Autodesk Fusion 360 part; units mm, degrees
(part 10 of 13)
  line L8044 (144.1, -138.589) -> (144.278, -138.571)
  line L8045 (144.602, -140.099) -> (144.433, -140.154)
  line L8046 (143.779, -138.74) -> (143.931, -138.647)
  line L8047 (118.974, -133.265) -> (118.977, -133.268)
  line L8048 (121.742, -140.099) -> (121.573, -140.154)
  line L8049 (119.499, -138.874) -> (119.593, -139.025)
  line L8050 (118.238, -139.859) -> (118.146, -139.706)
  line L8051 (118.252, -138.865) -> (118.379, -138.74)
  line L8052 (118.747, -133.387) -> (117.468, -132.108)
  line L8053 (117.291, -132.155) -> (117.168, -132.135)
  line L8054 (121.573, -140.154) -> (121.395, -140.17)
  line L8055 (122.212, -139.371) -> (122.212, -139.393)
  line L8056 (118.747, -138.584) -> (118.747, -133.387)
  line L8057 (119.356, -140.008) -> (119.202, -140.099)
  line L8058 (116.891, -131.755) -> (116.911, -131.631)
  line L8059 (119.223, -138.652) -> (119.373, -138.747)
  line L8060 (117.056, -131.431) -> (117.168, -131.374)
  line L8061 (117.415, -132.135) -> (117.291, -132.155)
  line L8062 (118.7, -138.589) -> (118.747, -138.584)
  line L8063 (119.485, -139.885) -> (119.356, -140.008)
  line L8064 (119.672, -139.371) -> (119.672, -139.393)
  line L8065 (118.072, -139.359) -> (118.094, -139.182)
  line L8066 (119.652, -139.193) -> (119.672, -139.371)
  line L8067 (119.033, -140.154) -> (118.855, -140.17)
  line L8068 (116.968, -131.52) -> (117.056, -131.431)
  line L8069 (121.595, -138.592) -> (121.763, -138.652)
  line L8070 (119.373, -138.747) -> (119.499, -138.874)
  line L8071 (119.202, -140.099) -> (119.033, -140.154)
  line L8072 (121.218, -140.147) -> (121.051, -140.085)
  line L8073 (122.124, -139.736) -> (122.025, -139.885)
  line L8074 (116.911, -131.878) -> (116.891, -131.755)
  line L8075 (118.379, -138.74) -> (118.531, -138.647)
  line L8076 (120.902, -139.987) -> (120.778, -139.859)
  line L8077 (117.168, -132.135) -> (117.056, -132.078)
  line L8078 (118.997, -133.336) -> (118.997, -138.585)
  line L8079 (118.997, -138.585) -> (119.055, -138.592)
  line L8080 (121.763, -138.652) -> (121.913, -138.747)
  line L8081 (119.055, -138.592) -> (119.223, -138.652)
  line L8082 (119.647, -139.57) -> (119.584, -139.736)
  line L8083 (121.913, -138.747) -> (122.039, -138.874)
  line L8084 (121.896, -140.008) -> (121.742, -140.099)
  line L8085 (117.291, -131.355) -> (117.415, -131.374)
  line L8086 (117.468, -132.108) -> (117.415, -132.135)
  line L8087 (118.362, -139.987) -> (118.238, -139.859)
  line L8088 (121.051, -140.085) -> (120.902, -139.987)
  line L8089 (117.168, -131.374) -> (117.291, -131.355)
  line L8090 (122.039, -138.874) -> (122.133, -139.025)
  line L8091 (121.395, -140.17) -> (121.218, -140.147)
  line L8092 (116.911, -131.631) -> (116.968, -131.52)
  line L8093 (122.187, -139.57) -> (122.124, -139.736)
  line L8094 (122.212, -139.393) -> (122.187, -139.57)
  line L8095 (119.584, -139.736) -> (119.485, -139.885)
  line L8096 (136.835, -138.592) -> (137.003, -138.652)
  line L8097 (120.629, -139.537) -> (120.612, -139.359)
  line L8098 (121.24, -138.589) -> (121.418, -138.571)
  line L8099 (136.813, -140.154) -> (136.635, -140.17)
  line L8100 (123.152, -139.359) -> (123.174, -139.182)
  line L8101 (123.318, -139.859) -> (123.226, -139.706)
  line L8102 (136.458, -140.147) -> (136.291, -140.085)
  line L8103 (123.174, -139.182) -> (123.235, -139.015)
  line L8104 (124.135, -138.592) -> (124.303, -138.652)
  line L8105 (135.926, -139.706) -> (135.869, -139.537)
  line L8106 (124.664, -139.736) -> (124.565, -139.885)
  line L8107 (137.364, -139.736) -> (137.265, -139.885)
  line L8108 (136.018, -139.859) -> (135.926, -139.706)
  line L8109 (122.192, -139.193) -> (122.212, -139.371)
  line L8110 (137.279, -138.874) -> (137.373, -139.025)
  line L8111 (123.169, -139.537) -> (123.152, -139.359)
  line L8112 (135.935, -139.015) -> (136.032, -138.865)
  line L8113 (124.113, -140.154) -> (123.935, -140.17)
  line L8114 (124.752, -139.393) -> (124.727, -139.57)
  line L8115 (120.612, -139.359) -> (120.634, -139.182)
  line L8116 (137.432, -139.193) -> (137.452, -139.371)
  line L8117 (120.634, -139.182) -> (120.695, -139.015)
  line L8118 (137.265, -139.885) -> (137.136, -140.008)
  line L8119 (123.235, -139.015) -> (123.332, -138.865)
  line L8120 (124.673, -139.025) -> (124.732, -139.193)
  line L8121 (120.792, -138.865) -> (120.919, -138.74)
  line L8122 (137.373, -139.025) -> (137.432, -139.193)
  line L8123 (137.136, -140.008) -> (136.982, -140.099)
  line L8124 (137.452, -139.393) -> (137.427, -139.57)
  line L8125 (137.003, -138.652) -> (137.153, -138.747)
  line L8126 (120.686, -139.706) -> (120.629, -139.537)
  line L8127 (136.982, -140.099) -> (136.813, -140.154)
  line L8128 (136.142, -139.987) -> (136.018, -139.859)
  line L8129 (137.153, -138.747) -> (137.279, -138.874)
  line L8130 (117.056, -132.078) -> (116.968, -131.99)
  line L8131 (137.427, -139.57) -> (137.364, -139.736)
  line L8132 (120.778, -139.859) -> (120.686, -139.706)
  line L8133 (137.452, -139.371) -> (137.452, -139.393)
  line L8134 (116.968, -131.99) -> (116.911, -131.878)
  line L8135 (120.919, -138.74) -> (121.071, -138.647)
  line L8136 (122.025, -139.885) -> (121.896, -140.008)
  line L8137 (121.418, -138.571) -> (121.595, -138.592)
  line L8138 (122.133, -139.025) -> (122.192, -139.193)
  line L8139 (135.869, -139.537) -> (135.852, -139.359)
  line L8140 (136.291, -140.085) -> (136.142, -139.987)
  line L8141 (121.071, -138.647) -> (121.24, -138.589)
  line L8142 (136.635, -140.17) -> (136.458, -140.147)
  line L8143 (120.695, -139.015) -> (120.792, -138.865)
  line L8144 (124.303, -138.652) -> (124.453, -138.747)
  line L8145 (127.119, -138.874) -> (127.213, -139.025)
  line L8146 (125.766, -139.706) -> (125.709, -139.537)
  line L8147 (124.453, -138.747) -> (124.579, -138.874)
  line L8148 (124.579, -138.874) -> (124.673, -139.025)
  line L8149 (136.658, -138.571) -> (136.835, -138.592)
  line L8150 (123.442, -139.987) -> (123.318, -139.859)
  line L8151 (124.752, -139.371) -> (124.752, -139.393)
  line L8152 (127.204, -139.736) -> (127.105, -139.885)
  line L8153 (127.292, -139.393) -> (127.267, -139.57)
  line L8154 (126.843, -138.652) -> (126.993, -138.747)
  line L8155 (136.159, -138.74) -> (136.311, -138.647)
  line L8156 (135.852, -139.359) -> (135.874, -139.182)
  line L8157 (125.999, -138.74) -> (126.151, -138.647)
  line L8158 (123.459, -138.74) -> (123.611, -138.647)
  line L8159 (126.822, -140.099) -> (126.653, -140.154)
  line L8160 (126.653, -140.154) -> (126.475, -140.17)
  line L8161 (126.151, -138.647) -> (126.32, -138.589)
  line L8162 (126.475, -140.17) -> (126.298, -140.147)
  line L8163 (136.48, -138.589) -> (136.658, -138.571)
  line L8164 (136.311, -138.647) -> (136.48, -138.589)
  line L8165 (123.935, -140.17) -> (123.758, -140.147)
  line L8166 (124.282, -140.099) -> (124.113, -140.154)
  line L8167 (136.032, -138.865) -> (136.159, -138.74)
  line L8168 (123.758, -140.147) -> (123.591, -140.085)
  line L8169 (125.692, -139.359) -> (125.714, -139.182)
  line L8170 (125.872, -138.865) -> (125.999, -138.74)
  line L8171 (127.272, -139.193) -> (127.292, -139.371)
  line L8172 (126.131, -140.085) -> (125.982, -139.987)
  line L8173 (123.226, -139.706) -> (123.169, -139.537)
  line L8174 (124.727, -139.57) -> (124.664, -139.736)
  line L8175 (123.332, -138.865) -> (123.459, -138.74)
  line L8176 (126.976, -140.008) -> (126.822, -140.099)
  line L8177 (125.714, -139.182) -> (125.775, -139.015)
  line L8178 (124.436, -140.008) -> (124.282, -140.099)
  line L8179 (123.611, -138.647) -> (123.78, -138.589)
  line L8180 (126.298, -140.147) -> (126.131, -140.085)
  line L8181 (125.982, -139.987) -> (125.858, -139.859)
  line L8182 (125.858, -139.859) -> (125.766, -139.706)
  line L8183 (125.775, -139.015) -> (125.872, -138.865)
  line L8184 (124.732, -139.193) -> (124.752, -139.371)
  line L8185 (127.292, -139.371) -> (127.292, -139.393)
  line L8186 (126.675, -138.592) -> (126.843, -138.652)
  line L8187 (123.958, -138.571) -> (124.135, -138.592)
  line L8188 (135.874, -139.182) -> (135.935, -139.015)
  line L8189 (124.565, -139.885) -> (124.436, -140.008)
  line L8190 (123.78, -138.589) -> (123.958, -138.571)
  line L8191 (123.591, -140.085) -> (123.442, -139.987)
  line L8192 (115.822, -139.987) -> (115.698, -139.859)
  line L8193 (131.755, -138.592) -> (131.923, -138.652)
  line L8194 (115.698, -139.859) -> (115.606, -139.706)
  line L8195 (116.493, -140.154) -> (116.315, -140.17)
  line L8196 (126.993, -138.747) -> (127.119, -138.874)
  line L8197 (115.839, -138.74) -> (115.991, -138.647)
  line L8198 (116.338, -138.571) -> (116.515, -138.592)
  line L8199 (116.662, -140.099) -> (116.493, -140.154)
  line L8200 (125.709, -139.537) -> (125.692, -139.359)
  line L8201 (129.215, -138.592) -> (129.383, -138.652)
  line L8202 (116.515, -138.592) -> (116.683, -138.652)
  line L8203 (116.683, -138.652) -> (116.833, -138.747)
  line L8204 (116.315, -140.17) -> (116.138, -140.147)
  line L8205 (115.712, -138.865) -> (115.839, -138.74)
  line L8206 (127.267, -139.57) -> (127.204, -139.736)
  line L8207 (127.105, -139.885) -> (126.976, -140.008)
  line L8208 (126.498, -138.571) -> (126.675, -138.592)
  line L8209 (115.532, -139.359) -> (115.554, -139.182)
  line L8210 (117.112, -139.193) -> (117.132, -139.371)
  line L8211 (115.971, -140.085) -> (115.822, -139.987)
  line L8212 (116.833, -138.747) -> (116.959, -138.874)
  line L8213 (115.615, -139.015) -> (115.712, -138.865)
  line L8214 (115.549, -139.537) -> (115.532, -139.359)
  line L8215 (126.32, -138.589) -> (126.498, -138.571)
  line L8216 (115.991, -138.647) -> (116.16, -138.589)
  line L8217 (116.16, -138.589) -> (116.338, -138.571)
  line L8218 (129.753, -139.025) -> (129.812, -139.193)
  line L8219 (115.554, -139.182) -> (115.615, -139.015)
  line L8220 (117.132, -139.371) -> (117.132, -139.393)
  line L8221 (128.398, -139.859) -> (128.306, -139.706)
  line L8222 (128.315, -139.015) -> (128.412, -138.865)
  line L8223 (115.606, -139.706) -> (115.549, -139.537)
  line L8224 (117.044, -139.736) -> (116.945, -139.885)
  line L8225 (116.945, -139.885) -> (116.816, -140.008)
  line L8226 (116.816, -140.008) -> (116.662, -140.099)
  line L8227 (117.132, -139.393) -> (117.107, -139.57)
  line L8228 (129.193, -140.154) -> (129.015, -140.17)
  line L8229 (129.659, -138.874) -> (129.753, -139.025)
  line L8230 (117.107, -139.57) -> (117.044, -139.736)
  line L8231 (127.213, -139.025) -> (127.272, -139.193)
  line L8232 (129.744, -139.736) -> (129.645, -139.885)
  line L8233 (116.959, -138.874) -> (117.053, -139.025)
  line L8234 (128.691, -138.647) -> (128.86, -138.589)
  line L8235 (117.053, -139.025) -> (117.112, -139.193)
  line L8236 (128.86, -138.589) -> (129.038, -138.571)
  line L8237 (129.832, -139.393) -> (129.807, -139.57)
  line L8238 (116.138, -140.147) -> (115.971, -140.085)
  line L8239 (129.038, -138.571) -> (129.215, -138.592)
  line L8240 (131.555, -140.17) -> (131.378, -140.147)
  line L8241 (130.855, -139.015) -> (130.952, -138.865)
  line L8242 (132.199, -138.874) -> (132.293, -139.025)
  line L8243 (139.693, -138.747) -> (139.819, -138.874)
  line L8244 (132.284, -139.736) -> (132.185, -139.885)
  line L8245 (139.913, -139.025) -> (139.972, -139.193)
  line L8246 (129.015, -140.17) -> (128.838, -140.147)
  line L8247 (132.293, -139.025) -> (132.352, -139.193)
  line L8248 (129.812, -139.193) -> (129.832, -139.371)
  line L8249 (128.412, -138.865) -> (128.539, -138.74)
  line L8250 (128.232, -139.359) -> (128.254, -139.182)
  line L8251 (130.789, -139.537) -> (130.772, -139.359)
  line L8252 (128.249, -139.537) -> (128.232, -139.359)
  line L8253 (130.772, -139.359) -> (130.794, -139.182)
  line L8254 (131.902, -140.099) -> (131.733, -140.154)
  line L8255 (131.378, -140.147) -> (131.211, -140.085)
  line L8256 (129.645, -139.885) -> (129.516, -140.008)
  line L8257 (129.362, -140.099) -> (129.193, -140.154)
  line L8258 (139.992, -139.371) -> (139.992, -139.393)
  line L8259 (129.516, -140.008) -> (129.362, -140.099)
  line L8260 (132.372, -139.371) -> (132.372, -139.393)
  line L8261 (131.733, -140.154) -> (131.555, -140.17)
  line L8262 (128.671, -140.085) -> (128.522, -139.987)
  line L8263 (129.807, -139.57) -> (129.744, -139.736)
  line L8264 (128.306, -139.706) -> (128.249, -139.537)
  line L8265 (128.254, -139.182) -> (128.315, -139.015)
  line L8266 (139.543, -138.652) -> (139.693, -138.747)
  line L8267 (129.383, -138.652) -> (129.533, -138.747)
  line L8268 (131.923, -138.652) -> (132.073, -138.747)
  line L8269 (131.062, -139.987) -> (130.938, -139.859)
  line L8270 (131.231, -138.647) -> (131.4, -138.589)
  line L8271 (132.185, -139.885) -> (132.056, -140.008)
  line L8272 (132.352, -139.193) -> (132.372, -139.371)
  line L8273 (139.819, -138.874) -> (139.913, -139.025)
  line L8274 (130.846, -139.706) -> (130.789, -139.537)
  line L8275 (139.375, -138.592) -> (139.543, -138.652)
  line L8276 (132.347, -139.57) -> (132.284, -139.736)
  line L8277 (129.832, -139.371) -> (129.832, -139.393)
  line L8278 (128.522, -139.987) -> (128.398, -139.859)
  line L8279 (131.578, -138.571) -> (131.755, -138.592)
  line L8280 (128.838, -140.147) -> (128.671, -140.085)
  line L8281 (128.539, -138.74) -> (128.691, -138.647)
  line L8282 (132.073, -138.747) -> (132.199, -138.874)
  line L8283 (131.4, -138.589) -> (131.578, -138.571)
  line L8284 (129.533, -138.747) -> (129.659, -138.874)
  line L8285 (131.079, -138.74) -> (131.231, -138.647)
  line L8286 (132.056, -140.008) -> (131.902, -140.099)
  line L8287 (132.372, -139.393) -> (132.347, -139.57)
  line L8288 (139.522, -140.099) -> (139.353, -140.154)
  line L8289 (142.359, -138.874) -> (142.453, -139.025)
  line L8290 (139.198, -138.571) -> (139.375, -138.592)
  line L8291 (142.512, -139.193) -> (142.532, -139.371)
  line L8292 (134.887, -139.57) -> (134.824, -139.736)
  line L8293 (142.062, -140.099) -> (141.893, -140.154)
  line L8294 (141.239, -138.74) -> (141.391, -138.647)
  line L8295 (140.949, -139.537) -> (140.932, -139.359)
  line L8296 (142.216, -140.008) -> (142.062, -140.099)
  line L8297 (138.414, -139.182) -> (138.475, -139.015)
  line L8298 (142.507, -139.57) -> (142.444, -139.736)
  line L8299 (138.558, -139.859) -> (138.466, -139.706)
  line L8300 (141.006, -139.706) -> (140.949, -139.537)
  line L8301 (141.915, -138.592) -> (142.083, -138.652)
  line L8302 (130.952, -138.865) -> (131.079, -138.74)
  line L8303 (142.532, -139.371) -> (142.532, -139.393)
  line L8304 (139.992, -139.393) -> (139.967, -139.57)
  line L8305 (138.851, -138.647) -> (139.02, -138.589)
  line L8306 (138.466, -139.706) -> (138.409, -139.537)
  line L8307 (142.444, -139.736) -> (142.345, -139.885)
  line L8308 (138.475, -139.015) -> (138.572, -138.865)
  line L8309 (138.831, -140.085) -> (138.682, -139.987)
  line L8310 (130.938, -139.859) -> (130.846, -139.706)
  line L8311 (139.175, -140.17) -> (138.998, -140.147)
  line L8312 (140.932, -139.359) -> (140.954, -139.182)
  line L8313 (142.083, -138.652) -> (142.233, -138.747)
  line L8314 (139.967, -139.57) -> (139.904, -139.736)
  line L8315 (142.345, -139.885) -> (142.216, -140.008)
  line L8316 (134.596, -140.008) -> (134.442, -140.099)
  line L8317 (131.211, -140.085) -> (131.062, -139.987)
  line L8318 (138.699, -138.74) -> (138.851, -138.647)
  line L8319 (142.532, -139.393) -> (142.507, -139.57)
  line L8320 (134.442, -140.099) -> (134.273, -140.154)
  line L8321 (139.02, -138.589) -> (139.198, -138.571)
  line L8322 (141.538, -140.147) -> (141.371, -140.085)
  line L8323 (139.972, -139.193) -> (139.992, -139.371)
  line L8324 (142.453, -139.025) -> (142.512, -139.193)
  line L8325 (138.682, -139.987) -> (138.558, -139.859)
  line L8326 (139.805, -139.885) -> (139.676, -140.008)
  line L8327 (130.794, -139.182) -> (130.855, -139.015)
  line L8328 (139.353, -140.154) -> (139.175, -140.17)
  line L8329 (142.233, -138.747) -> (142.359, -138.874)
  line L8330 (139.676, -140.008) -> (139.522, -140.099)
  line L8331 (138.998, -140.147) -> (138.831, -140.085)
  line L8332 (139.904, -139.736) -> (139.805, -139.885)
  line L8333 (138.392, -139.359) -> (138.414, -139.182)
  line L8334 (138.572, -138.865) -> (138.699, -138.74)
  line L8335 (138.409, -139.537) -> (138.392, -139.359)
  line L8336 (141.715, -140.17) -> (141.538, -140.147)
  line L8337 (134.273, -140.154) -> (134.095, -140.17)
  line L8338 (133.751, -140.085) -> (133.602, -139.987)
  line L8339 (134.095, -140.17) -> (133.918, -140.147)
  line L8340 (147.533, -139.025) -> (147.592, -139.193)
  line L8341 (141.391, -138.647) -> (141.56, -138.589)
  line L8342 (141.56, -138.589) -> (141.738, -138.571)
  line L8343 (134.295, -138.592) -> (134.463, -138.652)
  line L8344 (147.142, -140.099) -> (146.973, -140.154)
  line L8345 (147.425, -139.885) -> (147.296, -140.008)
  line L8346 (146.995, -138.592) -> (147.163, -138.652)
  line L8347 (134.725, -139.885) -> (134.596, -140.008)
  line L8348 (134.912, -139.393) -> (134.887, -139.57)
  line L8349 (141.098, -139.859) -> (141.006, -139.706)
  line L8350 (146.973, -140.154) -> (146.795, -140.17)
  line L8351 (146.795, -140.17) -> (146.618, -140.147)
  line L8352 (133.312, -139.359) -> (133.334, -139.182)
  line L8353 (141.222, -139.987) -> (141.098, -139.859)
  line L8354 (147.587, -139.57) -> (147.524, -139.736)
  line L8355 (141.738, -138.571) -> (141.915, -138.592)
  line L8356 (134.833, -139.025) -> (134.892, -139.193)
  line L8357 (133.334, -139.182) -> (133.395, -139.015)
  line L8358 (134.613, -138.747) -> (134.739, -138.874)
  line L8359 (141.015, -139.015) -> (141.112, -138.865)
  line L8360 (147.296, -140.008) -> (147.142, -140.099)
  line L8361 (146.618, -140.147) -> (146.451, -140.085)
  line L8362 (147.524, -139.736) -> (147.425, -139.885)
  line L8363 (133.94, -138.589) -> (134.118, -138.571)
  line L8364 (133.395, -139.015) -> (133.492, -138.865)
  line L8365 (141.112, -138.865) -> (141.239, -138.74)
  line L8366 (147.439, -138.874) -> (147.533, -139.025)
  line L8367 (147.313, -138.747) -> (147.439, -138.874)
  line L8368 (133.478, -139.859) -> (133.386, -139.706)
  line L8369 (141.893, -140.154) -> (141.715, -140.17)
  line L8370 (134.463, -138.652) -> (134.613, -138.747)
  line L8371 (147.612, -139.371) -> (147.612, -139.393)
  line L8372 (134.118, -138.571) -> (134.295, -138.592)
  line L8373 (140.954, -139.182) -> (141.015, -139.015)
  line L8374 (134.892, -139.193) -> (134.912, -139.371)
  line L8375 (141.371, -140.085) -> (141.222, -139.987)
  line L8376 (134.739, -138.874) -> (134.833, -139.025)
  line L8377 (133.771, -138.647) -> (133.94, -138.589)
  line L8378 (134.824, -139.736) -> (134.725, -139.885)
  line L8379 (133.386, -139.706) -> (133.329, -139.537)
  line L8380 (133.619, -138.74) -> (133.771, -138.647)
  line L8381 (133.492, -138.865) -> (133.619, -138.74)
  line L8382 (147.163, -138.652) -> (147.313, -138.747)
  line L8383 (134.912, -139.371) -> (134.912, -139.393)
  line L8384 (143.75, -124.929) -> (143.732, -124.943)
  line L8385 (146.086, -122.026) -> (146.029, -121.857)
  line L8386 (143.726, -124.947) -> (143.721, -124.951)
  line L8387 (146.319, -138.74) -> (146.471, -138.647)
  line L8388 (147.612, -139.393) -> (147.587, -139.57)
  line L8389 (105.027, -122.529) -> (107.214, -124.716)
  line L8390 (146.818, -138.571) -> (146.995, -138.592)
  line L8391 (105.744, -119.532) -> (105.691, -119.505)
  line L8392 (146.64, -138.589) -> (146.818, -138.571)
  line L8393 (146.471, -138.647) -> (146.64, -138.589)
  line L8394 (107.214, -124.716) -> (143.61, -124.716)
  line L8395 (105.867, -119.551) -> (105.744, -119.532)
  line L8396 (106.191, -119.387) -> (106.102, -119.475)
  line L8397 (147.592, -139.193) -> (147.612, -139.371)
  line L8398 (106.248, -119.275) -> (106.191, -119.387)
  line L8399 (105.991, -118.771) -> (106.102, -118.828)
  line L8400 (146.012, -139.359) -> (146.034, -139.182)
  line L8401 (106.267, -119.151) -> (106.248, -119.275)
  line L8402 (106.248, -119.028) -> (106.267, -119.151)
  line L8403 (133.918, -140.147) -> (133.751, -140.085)
  line L8404 (146.086, -139.706) -> (146.029, -139.537)
  line L8405 (146.166, -122.159) -> (146.086, -122.026)
  line L8406 (146.034, -139.182) -> (146.095, -139.015)
  line L8407 (146.178, -139.859) -> (146.086, -139.706)
  line L8408 (146.029, -121.857) -> (146.012, -121.679)
  line L8409 (106.102, -119.475) -> (105.991, -119.532)
  line L8410 (105.027, -120.168) -> (105.027, -122.529)
  line L8411 (146.451, -122.405) -> (146.345, -122.335)
  line L8412 (146.64, -120.909) -> (146.818, -120.891)
  line L8413 (106.102, -118.828) -> (106.191, -118.916)
  line L8414 (105.991, -119.532) -> (105.867, -119.551)
  line L8415 (146.192, -121.185) -> (146.319, -121.06)
  line L8416 (146.029, -139.537) -> (146.012, -139.359)
  line L8417 (146.095, -139.015) -> (146.192, -138.865)
  line L8418 (146.451, -140.085) -> (146.302, -139.987)
  line L8419 (143.61, -124.716) -> (146.166, -122.159)
  line L8420 (147.612, -121.713) -> (147.587, -121.89)
  line L8421 (146.618, -122.467) -> (146.451, -122.405)
  line L8422 (133.602, -139.987) -> (133.478, -139.859)
  line L8423 (146.302, -139.987) -> (146.178, -139.859)
  line L8424 (147.612, -121.691) -> (147.612, -121.713)
  line L8425 (105.691, -119.505) -> (105.027, -120.168)
  line L8426 (133.329, -139.537) -> (133.312, -139.359)
  line L8427 (146.192, -138.865) -> (146.319, -138.74)
  line L8428 (106.191, -118.916) -> (106.248, -119.028)
  line L8429 (146.795, -122.49) -> (146.618, -122.467)
  line L8430 (146.319, -121.06) -> (146.471, -120.967)
  line L8431 (147.587, -121.89) -> (147.524, -122.056)
  line L8432 (104.78, -120.09) -> (104.781, -120.087)
  line L8433 (143.729, -124.946) -> (143.726, -124.947)
  line L8434 (107.127, -124.961) -> (107.101, -124.944)
  line L8435 (143.626, -122.159) -> (143.546, -122.026)
  line L8436 (107.074, -124.929) -> (104.814, -122.669)
  line L8437 (104.777, -122.58) -> (104.777, -120.117)
  line L8438 (146.034, -121.502) -> (146.095, -121.335)
  line L8439 (146.012, -121.679) -> (146.034, -121.502)
  line L8440 (104.814, -120.028) -> (105.514, -119.328)
  line L8441 (143.721, -124.951) -> (143.691, -124.957)
  line L8442 (147.592, -121.513) -> (147.612, -121.691)
  line L8443 (147.142, -122.419) -> (146.973, -122.474)
  line L8444 (147.163, -120.972) -> (147.313, -121.067)
  line L8445 (143.546, -122.026) -> (143.489, -121.857)
  line L8446 (105.544, -118.916) -> (105.632, -118.828)
  line L8447 (104.814, -122.669) -> (104.8, -122.651)
  line L8448 (104.796, -122.645) -> (104.792, -122.64)
  line L8449 (107.136, -124.963) -> (107.133, -124.962)
  line L8450 (146.345, -122.335) -> (143.75, -124.929)
  line L8451 (146.818, -120.891) -> (146.995, -120.912)
  line L8452 (147.439, -121.194) -> (147.533, -121.345)
  line L8453 (146.471, -120.967) -> (146.64, -120.909)
  line L8454 (104.792, -122.64) -> (104.786, -122.61)
  line L8455 (104.799, -120.055) -> (104.814, -120.028)
  line L8456 (146.995, -120.912) -> (147.163, -120.972)
  line L8457 (147.533, -121.345) -> (147.592, -121.513)
  line L8458 (143.732, -124.943) -> (143.729, -124.946)
  line L8459 (105.744, -118.771) -> (105.867, -118.751)
  line L8460 (104.786, -122.61) -> (104.777, -122.58)
  line L8461 (104.781, -120.087) -> (104.782, -120.081)
  line L8462 (104.782, -120.081) -> (104.799, -120.055)
  line L8463 (147.313, -121.067) -> (147.439, -121.194)
  line L8464 (105.867, -118.751) -> (105.991, -118.771)
  line L8465 (104.797, -122.648) -> (104.796, -122.645)
  line L8466 (143.662, -124.966) -> (107.163, -124.966)
  line L8467 (146.095, -121.335) -> (146.192, -121.185)
  line L8468 (107.163, -124.966) -> (107.141, -124.963)
  line L8469 (105.487, -119.275) -> (105.467, -119.151)
  line L8470 (107.101, -124.944) -> (107.074, -124.929)
  line L8471 (104.78, -120.095) -> (104.78, -120.09)
  line L8472 (104.777, -120.117) -> (104.78, -120.095)
  line L8473 (105.514, -119.328) -> (105.487, -119.275)
  line L8474 (146.973, -122.474) -> (146.795, -122.49)
  line L8475 (147.425, -122.205) -> (147.296, -122.328)
  line L8476 (104.8, -122.651) -> (104.797, -122.648)
  line L8477 (147.524, -122.056) -> (147.425, -122.205)
  line L8478 (143.691, -124.957) -> (143.662, -124.966)
  line L8479 (147.296, -122.328) -> (147.142, -122.419)
  line L8480 (145.052, -121.513) -> (145.072, -121.691)
  line L8481 (143.555, -121.335) -> (143.652, -121.185)
  line L8482 (144.1, -120.909) -> (144.278, -120.891)
  line L8483 (107.061, -117.278) -> (107.185, -117.298)
  line L8484 (143.931, -120.967) -> (144.1, -120.909)
  line L8485 (107.462, -122.827) -> (107.462, -118.256)
  line L8486 (107.061, -118.078) -> (106.937, -118.059)
  line L8487 (106.937, -118.059) -> (106.826, -118.002)
  line L8488 (144.602, -122.419) -> (144.433, -122.474)
  line L8489 (107.482, -122.895) -> (107.481, -122.892)
  line L8490 (143.489, -121.857) -> (143.472, -121.679)
  line L8491 (107.133, -124.962) -> (107.127, -124.961)
  line L8492 (141.878, -124.257) -> (141.875, -124.26)
  line L8493 (143.805, -122.335) -> (141.896, -124.244)
  line L8494 (145.047, -121.89) -> (144.984, -122.056)
  line L8495 (107.185, -118.059) -> (107.061, -118.078)
  line L8496 (143.494, -121.502) -> (143.555, -121.335)
  line L8497 (108.854, -124.258) -> (108.827, -124.244)
  line L8498 (144.433, -122.474) -> (144.255, -122.49)
  line L8499 (141.872, -124.261) -> (141.867, -124.265)
  line L8500 (141.807, -124.28) -> (108.915, -124.28)
  line L8501 (144.078, -122.467) -> (143.911, -122.405)
  line L8502 (106.826, -118.002) -> (106.737, -117.913)
  line L8503 (105.487, -119.028) -> (105.544, -118.916)
  line L8504 (107.141, -124.963) -> (107.136, -124.963)
  line L8505 (143.652, -121.185) -> (143.779, -121.06)
  line L8506 (145.072, -121.691) -> (145.072, -121.713)
  line L8507 (144.899, -121.194) -> (144.993, -121.345)
  line L8508 (144.623, -120.972) -> (144.773, -121.067)
  line L8509 (145.072, -121.713) -> (145.047, -121.89)
  line L8510 (143.911, -122.405) -> (143.805, -122.335)
  line L8511 (141.875, -124.26) -> (141.872, -124.261)
  line L8512 (144.455, -120.912) -> (144.623, -120.972)
  line L8513 (144.993, -121.345) -> (145.052, -121.513)
  line L8514 (107.485, -122.898) -> (107.482, -122.895)
  line L8515 (141.896, -124.244) -> (141.878, -124.257)
  line L8516 (105.632, -118.828) -> (105.744, -118.771)
  line L8517 (144.255, -122.49) -> (144.078, -122.467)
  line L8518 (105.467, -119.151) -> (105.487, -119.028)
  line L8519 (143.472, -121.679) -> (143.494, -121.502)
  line L8520 (144.278, -120.891) -> (144.455, -120.912)
  line L8521 (144.885, -122.205) -> (144.756, -122.328)
  line L8522 (144.756, -122.328) -> (144.602, -122.419)
  line L8523 (141.867, -124.265) -> (141.837, -124.272)
  line L8524 (144.984, -122.056) -> (144.885, -122.205)
  line L8525 (143.779, -121.06) -> (143.931, -120.967)
  line L8526 (108.893, -124.277) -> (108.889, -124.277)
  line L8527 (144.773, -121.067) -> (144.899, -121.194)
  line L8528 (129.872, -138.361) -> (129.719, -138.254)
  line L8529 (127.876, -138.753) -> (127.829, -138.806)
  line L8530 (128.804, -138.077) -> (128.799, -138.078)
  line L8531 (130.732, -138.361) -> (130.728, -138.364)
  line L8532 (129.26, -138.077) -> (129.032, -138.057)
  line L8533 (128.799, -138.078) -> (128.588, -138.135)
  line L8534 (129.719, -138.254) -> (129.689, -138.233)
  line L8535 (128.588, -138.135) -> (128.583, -138.136)
  line L8536 (127.892, -138.719) -> (127.876, -138.753)
  line L8537 (127.648, -138.753) -> (127.632, -138.719)
  line L8538 (129.481, -138.136) -> (129.476, -138.135)
  line L8539 (130.188, -138.753) -> (130.172, -138.719)
  line L8540 (127.894, -138.714) -> (127.892, -138.719)
  line L8541 (128.578, -138.139) -> (128.38, -138.231)
  line L8542 (128.583, -138.136) -> (128.578, -138.139)
  line L8543 (128.375, -138.233) -> (128.345, -138.254)
  line L8544 (129.265, -138.078) -> (129.26, -138.077)
  line L8545 (130.885, -138.254) -> (130.732, -138.361)
  line L8546 (130.432, -138.719) -> (130.416, -138.753)
  line L8547 (129.689, -138.233) -> (129.684, -138.231)
  line L8548 (129.032, -138.057) -> (128.804, -138.077)
  line L8549 (127.632, -138.719) -> (127.632, -138.719)
  line L8550 (130.566, -138.526) -> (130.434, -138.714)
  line L8551 (130.915, -138.233) -> (130.885, -138.254)
  line L8552 (130.732, -138.361) -> (130.732, -138.361)
  line L8553 (130.728, -138.364) -> (130.566, -138.526)
  line L8554 (128.588, -138.135) -> (128.588, -138.135)
  line L8555 (129.476, -138.135) -> (129.265, -138.078)
  line L8556 (128.188, -138.364) -> (128.026, -138.526)
  line L8557 (130.17, -138.714) -> (130.038, -138.526)
  line L8558 (127.693, -138.805) -> (127.648, -138.753)
  line L8559 (127.829, -138.806) -> (127.761, -138.826)
  line L8560 (128.026, -138.526) -> (127.894, -138.714)
  line L8561 (130.92, -138.231) -> (130.92, -138.231)
  line L8562 (128.38, -138.231) -> (128.38, -138.231)
  line L8563 (128.192, -138.361) -> (128.192, -138.361)
  line L8564 (130.92, -138.231) -> (130.915, -138.233)
  line L8565 (129.265, -138.078) -> (129.265, -138.078)
  line L8566 (128.578, -138.139) -> (128.578, -138.139)
  line L8567 (128.345, -138.254) -> (128.192, -138.361)
  line L8568 (127.892, -138.719) -> (127.892, -138.719)
  line L8569 (127.632, -138.719) -> (127.63, -138.714)
  line L8570 (128.799, -138.078) -> (128.799, -138.078)
  line L8571 (130.172, -138.719) -> (130.172, -138.719)
  line L8572 (130.432, -138.719) -> (130.432, -138.719)
  line L8573 (129.486, -138.139) -> (129.481, -138.136)
  line L8574 (128.38, -138.231) -> (128.375, -138.233)
  line L8575 (128.192, -138.361) -> (128.188, -138.364)
  line L8576 (125.092, -138.719) -> (125.092, -138.719)
  line L8577 (124.792, -138.361) -> (124.792, -138.361)
  line L8578 (125.352, -138.719) -> (125.336, -138.753)
  line L8579 (126.259, -138.078) -> (126.259, -138.078)
  line L8580 (126.264, -138.077) -> (126.259, -138.078)
  line L8581 (126.048, -138.135) -> (126.048, -138.135)
  line L8582 (126.043, -138.136) -> (126.038, -138.139)
  line L8583 (125.652, -138.361) -> (125.648, -138.364)
  line L8584 (125.84, -138.231) -> (125.84, -138.231)
  line L8585 (124.796, -138.364) -> (124.792, -138.361)
  line L8586 (125.092, -138.719) -> (125.09, -138.714)
  line L8587 (127.63, -138.714) -> (127.498, -138.526)
  line L8588 (127.336, -138.364) -> (127.332, -138.361)
  line L8589 (126.72, -138.077) -> (126.492, -138.057)
  line L8590 (126.936, -138.135) -> (126.725, -138.078)
  line L8591 (125.835, -138.233) -> (125.805, -138.254)
  line L8592 (127.149, -138.233) -> (127.144, -138.231)
  line L8593 (126.936, -138.135) -> (126.936, -138.135)
  line L8594 (127.144, -138.231) -> (127.144, -138.231)
  line L8595 (127.144, -138.231) -> (126.946, -138.139)
  line L8596 (127.498, -138.526) -> (127.336, -138.364)
  line L8597 (126.048, -138.135) -> (126.043, -138.136)
  line L8598 (126.946, -138.139) -> (126.941, -138.136)
  line L8599 (125.648, -138.364) -> (125.486, -138.526)
  line L8600 (125.09, -138.714) -> (124.958, -138.526)
  line L8601 (124.604, -138.231) -> (124.406, -138.139)
  line L8602 (125.84, -138.231) -> (125.835, -138.233)
  line L8603 (126.941, -138.136) -> (126.936, -138.135)
  line L8604 (124.406, -138.139) -> (124.406, -138.139)
  line L8605 (125.336, -138.753) -> (125.289, -138.806)
  line L8606 (126.725, -138.078) -> (126.725, -138.078)
  line L8607 (124.396, -138.135) -> (124.396, -138.135)
  line L8608 (127.332, -138.361) -> (127.332, -138.361)
  line L8609 (127.179, -138.254) -> (127.149, -138.233)
  line L8610 (127.332, -138.361) -> (127.179, -138.254)
  line L8611 (127.761, -138.826) -> (127.693, -138.805)
  line L8612 (126.259, -138.078) -> (126.048, -138.135)
  line L8613 (126.946, -138.139) -> (126.946, -138.139)
  line L8614 (126.038, -138.139) -> (126.038, -138.139)
  line L8615 (125.652, -138.361) -> (125.652, -138.361)
  line L8616 (125.805, -138.254) -> (125.652, -138.361)
  line L8617 (126.725, -138.078) -> (126.72, -138.077)
  line L8618 (129.476, -138.135) -> (129.476, -138.135)
  line L8619 (124.185, -138.078) -> (124.185, -138.078)
  line L8620 (124.792, -138.361) -> (124.639, -138.254)
  line L8621 (125.486, -138.526) -> (125.354, -138.714)
  line L8622 (126.038, -138.139) -> (125.84, -138.231)
  line L8623 (126.492, -138.057) -> (126.264, -138.077)
  line L8624 (125.289, -138.806) -> (125.221, -138.826)
  line L8625 (124.958, -138.526) -> (124.796, -138.364)
  line L8626 (125.354, -138.714) -> (125.352, -138.719)
  line L8627 (125.153, -138.805) -> (125.108, -138.753)
  line L8628 (122.681, -138.826) -> (122.613, -138.805)
  line L8629 (125.108, -138.753) -> (125.092, -138.719)
  line L8630 (122.552, -138.719) -> (122.55, -138.714)
  line L8631 (123.3, -138.231) -> (123.3, -138.231)
  line L8632 (123.112, -138.361) -> (123.112, -138.361)
  line L8633 (122.55, -138.714) -> (122.418, -138.526)
  line L8634 (122.946, -138.526) -> (122.814, -138.714)
  line L8635 (122.099, -138.254) -> (122.069, -138.233)
  line L8636 (123.508, -138.135) -> (123.503, -138.136)
  line L8637 (124.18, -138.077) -> (123.952, -138.057)
  line L8638 (124.609, -138.233) -> (124.604, -138.231)
  line L8639 (122.256, -138.364) -> (122.252, -138.361)
  line L8640 (123.508, -138.135) -> (123.508, -138.135)
  line L8641 (122.749, -138.806) -> (122.681, -138.826)
  line L8642 (122.418, -138.526) -> (122.256, -138.364)
  line L8643 (122.613, -138.805) -> (122.568, -138.753)
  line L8644 (122.064, -138.231) -> (122.064, -138.231)
  line L8645 (123.3, -138.231) -> (123.295, -138.233)
  line L8646 (123.295, -138.233) -> (123.265, -138.254)
  line L8647 (124.406, -138.139) -> (124.401, -138.136)
  line L8648 (123.724, -138.077) -> (123.719, -138.078)
  line L8649 (125.352, -138.719) -> (125.352, -138.719)
  line L8650 (124.396, -138.135) -> (124.185, -138.078)
  line L8651 (123.719, -138.078) -> (123.719, -138.078)
  line L8652 (123.952, -138.057) -> (123.724, -138.077)
  line L8653 (124.639, -138.254) -> (124.609, -138.233)
  line L8654 (124.604, -138.231) -> (124.604, -138.231)
  line L8655 (123.498, -138.139) -> (123.498, -138.139)
  line L8656 (123.719, -138.078) -> (123.508, -138.135)
  line L8657 (123.498, -138.139) -> (123.3, -138.231)
  line L8658 (122.814, -138.714) -> (122.812, -138.719)
  line L8659 (123.108, -138.364) -> (122.946, -138.526)
  line L8660 (122.812, -138.719) -> (122.812, -138.719)
  line L8661 (123.265, -138.254) -> (123.112, -138.361)
  line L8662 (123.503, -138.136) -> (123.498, -138.139)
  line L8663 (124.185, -138.078) -> (124.18, -138.077)
  line L8664 (122.796, -138.753) -> (122.749, -138.806)
  line L8665 (122.252, -138.361) -> (122.099, -138.254)
  line L8666 (122.069, -138.233) -> (122.064, -138.231)
  line L8667 (123.112, -138.361) -> (123.108, -138.364)
  line L8668 (125.221, -138.826) -> (125.153, -138.805)
  line L8669 (122.252, -138.361) -> (122.252, -138.361)
  line L8670 (124.401, -138.136) -> (124.396, -138.135)
  line L8671 (122.812, -138.719) -> (122.796, -138.753)
  line L8672 (121.179, -138.078) -> (121.179, -138.078)
  line L8673 (119.515, -138.199) -> (119.505, -138.151)
  line L8674 (121.412, -138.057) -> (121.184, -138.077)
  line L8675 (120.406, -138.526) -> (120.274, -138.714)
  line L8676 (121.866, -138.139) -> (121.861, -138.136)
  line L8677 (121.861, -138.136) -> (121.856, -138.135)
  line L8678 (120.141, -138.826) -> (120.073, -138.805)
  line L8679 (120.968, -138.135) -> (120.963, -138.136)
  line L8680 (120.572, -138.361) -> (120.568, -138.364)
  line L8681 (119.559, -138.254) -> (119.515, -138.199)
  line L8682 (120.272, -138.719) -> (120.272, -138.719)
  line L8683 (120.725, -138.254) -> (120.572, -138.361)
  line L8684 (121.856, -138.135) -> (121.856, -138.135)
  line L8685 (120.073, -138.805) -> (120.028, -138.753)
  line L8686 (119.505, -138.151) -> (119.505, -133.414)
  line L8687 (119.505, -133.296) -> (119.505, -133.292)
  line L8688 (120.012, -138.719) -> (120.01, -138.714)
  line L8689 (119.505, -133.414) -> (119.506, -133.403)
  line L8690 (119.508, -133.396) -> (119.506, -133.328)
  line L8691 (120.01, -138.714) -> (119.878, -138.526)
  line L8692 (119.878, -138.526) -> (119.716, -138.364)
  line L8693 (120.76, -138.231) -> (120.76, -138.231)
  line L8694 (121.645, -138.078) -> (121.64, -138.077)
  line L8695 (120.958, -138.139) -> (120.76, -138.231)
  line L8696 (120.958, -138.139) -> (120.958, -138.139)
  line L8697 (120.963, -138.136) -> (120.958, -138.139)
  line L8698 (120.568, -138.364) -> (120.406, -138.526)
  line L8699 (120.968, -138.135) -> (120.968, -138.135)
  line L8700 (120.274, -138.714) -> (120.272, -138.719)
  line L8701 (122.064, -138.231) -> (121.866, -138.139)
  line L8702 (119.712, -138.361) -> (119.559, -138.254)
  line L8703 (122.552, -138.719) -> (122.552, -138.719)
  line L8704 (121.64, -138.077) -> (121.412, -138.057)
  line L8705 (119.488, -133.169) -> (119.488, -133.169)
  line L8706 (120.272, -138.719) -> (120.256, -138.753)
  line L8707 (120.256, -138.753) -> (120.209, -138.806)
  line L8708 (122.568, -138.753) -> (122.552, -138.719)
  line L8709 (121.866, -138.139) -> (121.866, -138.139)
  line L8710 (119.493, -133.197) -> (119.493, -133.196)
  line L8711 (120.028, -138.753) -> (120.012, -138.719)
  line L8712 (120.76, -138.231) -> (120.755, -138.233)
  line L8713 (121.179, -138.078) -> (120.968, -138.135)
  line L8714 (121.645, -138.078) -> (121.645, -138.078)
  line L8715 (121.856, -138.135) -> (121.645, -138.078)
  line L8716 (120.755, -138.233) -> (120.725, -138.254)
  line L8717 (120.209, -138.806) -> (120.141, -138.826)
  line L8718 (121.184, -138.077) -> (121.179, -138.078)
  line L8719 (120.572, -138.361) -> (120.572, -138.361)
  line L8720 (119.458, -133.082) -> (119.448, -133.065)
  line L8721 (119.342, -132.905) -> (119.337, -132.899)
  line L8722 (118.185, -131.565) -> (118.126, -131.383)
  line L8723 (119.716, -138.364) -> (119.712, -138.361)
  line L8724 (119.46, -133.09) -> (119.458, -133.082)
  line L8725 (119.506, -133.403) -> (119.508, -133.396)
  line L8726 (119.505, -133.324) -> (119.505, -133.296)
  line L8727 (120.012, -138.719) -> (120.012, -138.719)
  line L8728 (119.503, -133.244) -> (119.503, -133.236)
  line L8729 (119.377, -132.944) -> (119.362, -132.93)
  line L8730 (119.406, -132.992) -> (119.399, -132.982)
  line L8731 (117.393, -130.848) -> (117.393, -130.848)
  line L8732 (117.573, -130.886) -> (117.48, -130.866)
  line L8733 (119.362, -132.93) -> (119.349, -132.915)
  line L8734 (117.748, -130.964) -> (117.742, -130.961)
  line L8735 (118.126, -131.383) -> (118.03, -131.218)
  line L8736 (119.399, -132.982) -> (119.381, -132.951)
  line L8737 (119.432, -133.028) -> (119.406, -132.992)
  line L8738 (118.204, -131.744) -> (118.202, -131.73)
  line L8739 (118.185, -131.571) -> (118.185, -131.565)
  line L8740 (117.902, -131.076) -> (117.748, -130.964)
  line L8741 (118.03, -131.218) -> (117.902, -131.076)
  line L8742 (117.742, -130.961) -> (117.579, -130.889)
  line L8743 (117.579, -130.889) -> (117.579, -130.889)
  line L8744 (119.49, -133.177) -> (119.488, -133.169)
  line L8745 (119.712, -138.361) -> (119.712, -138.361)
  line L8746 (119.488, -133.169) -> (119.474, -133.136)
  line L8747 (119.505, -133.292) -> (119.504, -133.28)
  line L8748 (117.579, -130.889) -> (117.573, -130.886)
  line L8749 (119.439, -133.047) -> (119.434, -133.035)
  line L8750 (119.295, -132.862) -> (118.238, -131.806)
  line L8751 (118.238, -131.806) -> (118.204, -131.744)
  line L8752 (119.337, -132.899) -> (119.303, -132.87)
  line L8753 (119.381, -132.951) -> (119.377, -132.944)
  line L8754 (119.448, -133.065) -> (119.439, -133.047)
  line L8755 (119.503, -133.236) -> (119.497, -133.216)
  line L8756 (119.47, -133.124) -> (119.46, -133.09)
  line L8757 (117.742, -130.961) -> (117.742, -130.961)
  line L8758 (118.185, -131.571) -> (118.185, -131.571)
  line L8759 (119.349, -132.915) -> (119.342, -132.905)
  line L8760 (119.434, -133.035) -> (119.432, -133.028)
  line L8761 (119.504, -133.28) -> (119.503, -133.244)
  line L8762 (119.474, -133.136) -> (119.47, -133.124)
  line L8763 (119.493, -133.196) -> (119.49, -133.177)
  line L8764 (119.46, -133.09) -> (119.46, -133.09)
  line L8765 (119.497, -133.216) -> (119.493, -133.197)
  line L8766 (119.506, -133.328) -> (119.505, -133.324)
  line L8767 (117.48, -130.866) -> (117.393, -130.848)
  line L8768 (118.218, -138.219) -> (118.185, -138.254)
  line L8769 (117.102, -132.643) -> (117.189, -132.662)
  line L8770 (116.984, -138.231) -> (116.984, -138.231)
  line L8771 (116.378, -131.755) -> (116.398, -131.945)
  line L8772 (116.84, -132.549) -> (116.84, -132.549)
  line L8773 (116.552, -132.292) -> (116.68, -132.434)
  line L8774 (116.84, -132.549) -> (117.003, -132.621)
  line L8775 (116.834, -130.964) -> (116.68, -131.076)
  line L8776 (117.189, -132.662) -> (117.189, -132.662)
  line L8777 (118.032, -138.361) -> (118.028, -138.364)
  line L8778 (118.185, -138.254) -> (118.032, -138.361)
  line L8779 (117.172, -138.361) -> (117.172, -138.361)
  line L8780 (116.68, -132.434) -> (116.834, -132.546)
  line L8781 (118.202, -133.561) -> (118.236, -133.623)
  line L8782 (117.196, -130.846) -> (117.189, -130.848)
  line L8783 (117.189, -130.848) -> (117.189, -130.848)
  line L8784 (117.189, -132.662) -> (117.196, -132.663)
  line L8785 (117.252, -132.663) -> (117.32, -132.683)
  line L8786 (117.003, -130.889) -> (116.84, -130.961)
  line L8787 (117.189, -130.848) -> (117.102, -130.866)
  line L8788 (117.009, -130.886) -> (117.003, -130.889)
  line L8789 (117.102, -130.866) -> (117.009, -130.886)
  line L8790 (117.196, -132.663) -> (117.252, -132.663)
  line L8791 (116.552, -131.218) -> (116.457, -131.383)
  line L8792 (119.303, -132.87) -> (119.295, -132.862)
  line L8793 (117.003, -132.621) -> (117.009, -132.624)
  line L8794 (117.003, -130.889) -> (117.003, -130.889)
  line L8795 (116.84, -130.961) -> (116.84, -130.961)
  line L8796 (118.238, -138.151) -> (118.218, -138.219)
  line L8797 (116.457, -132.126) -> (116.552, -132.292)
  line L8798 (117.172, -138.361) -> (117.019, -138.254)
  line L8799 (117.019, -138.254) -> (116.989, -138.233)
  line L8800 (117.734, -138.714) -> (117.732, -138.719)
  line L8801 (118.202, -131.73) -> (118.185, -131.571)
  line L8802 (118.238, -133.65) -> (118.238, -138.151)
  line L8803 (116.84, -130.961) -> (116.834, -130.964)
  line L8804 (116.398, -131.945) -> (116.457, -132.126)
  line L8805 (117.393, -130.848) -> (117.387, -130.846)
  line L8806 (116.68, -131.076) -> (116.552, -131.218)
  line L8807 (116.398, -131.565) -> (116.378, -131.755)
  line L8808 (116.457, -131.383) -> (116.398, -131.565)
  line L8809 (117.32, -132.683) -> (117.341, -132.7)
  line L8810 (116.834, -132.546) -> (116.84, -132.549)
  line L8811 (117.387, -130.846) -> (117.196, -130.846)
  line L8812 (117.009, -132.624) -> (117.102, -132.643)
  line L8813 (118.236, -133.623) -> (118.238, -133.65)
  line L8814 (117.533, -138.805) -> (117.488, -138.753)
  line L8815 (117.472, -138.719) -> (117.47, -138.714)
  line L8816 (115.323, -138.531) -> (115.323, -138.531)
  line L8817 (115.488, -138.364) -> (115.326, -138.526)
  line L8818 (116.565, -138.078) -> (116.56, -138.077)
  line L8819 (115.015, -138.668) -> (114.926, -138.531)
  line L8820 (115.888, -138.135) -> (115.888, -138.135)
  line L8821 (116.781, -138.136) -> (116.776, -138.135)
  line L8822 (115.326, -138.526) -> (115.323, -138.531)
  line L8823 (117.488, -138.753) -> (117.472, -138.719)
  line L8824 (116.786, -138.139) -> (116.786, -138.139)
  line L8825 (117.338, -138.526) -> (117.176, -138.364)
  line L8826 (116.776, -138.135) -> (116.565, -138.078)
  line L8827 (115.68, -138.231) -> (115.675, -138.233)
  line L8828 (115.492, -138.361) -> (115.488, -138.364)
  line L8829 (117.866, -138.526) -> (117.734, -138.714)
  line L8830 (117.601, -138.826) -> (117.533, -138.805)
  line L8831 (115.883, -138.136) -> (115.878, -138.139)
  line L8832 (115.224, -138.672) -> (115.169, -138.716)
  line L8833 (116.565, -138.078) -> (116.565, -138.078)
  line L8834 (115.888, -138.135) -> (115.883, -138.136)
  line L8835 (116.776, -138.135) -> (116.776, -138.135)
  line L8836 (117.716, -138.753) -> (117.669, -138.806)
  line L8837 (114.926, -138.531) -> (114.912, -138.508)
  line L8838 (117.669, -138.806) -> (117.601, -138.826)
  line L8839 (116.989, -138.233) -> (116.984, -138.231)
  line L8840 (116.56, -138.077) -> (116.332, -138.057)
  line L8841 (115.169, -138.716) -> (115.098, -138.723)
  line L8842 (115.035, -138.691) -> (115.015, -138.668)
  line L8843 (116.104, -138.077) -> (116.099, -138.078)
  line L8844 (118.032, -138.361) -> (118.032, -138.361)
  line L8845 (117.47, -138.714) -> (117.338, -138.526)
  line L8846 (117.472, -138.719) -> (117.472, -138.719)
  line L8847 (114.912, -138.508) -> (114.892, -138.487)
  line L8848 (117.732, -138.719) -> (117.732, -138.719)
  line L8849 (116.099, -138.078) -> (116.099, -138.078)
  line L8850 (117.732, -138.719) -> (117.716, -138.753)
  line L8851 (117.341, -132.7) -> (118.202, -133.561)
  line L8852 (115.323, -138.531) -> (115.224, -138.672)
  line L8853 (115.878, -138.139) -> (115.68, -138.231)
  line L8854 (116.332, -138.057) -> (116.104, -138.077)
  line L8855 (115.68, -138.231) -> (115.68, -138.231)
  line L8856 (115.675, -138.233) -> (115.645, -138.254)
  line L8857 (115.878, -138.139) -> (115.878, -138.139)
  line L8858 (116.786, -138.139) -> (116.781, -138.136)
  line L8859 (117.176, -138.364) -> (117.172, -138.361)
  line L8860 (115.098, -138.723) -> (115.035, -138.691)
  line L8861 (115.645, -138.254) -> (115.492, -138.361)
  line L8862 (118.028, -138.364) -> (117.866, -138.526)
  line L8863 (116.984, -138.231) -> (116.786, -138.139)
  line L8864 (115.492, -138.361) -> (115.492, -138.361)
  line L8865 (113.925, -137.964) -> (113.852, -137.963)
  line L8866 (112.352, -138.487) -> (112.241, -138.364)
  line L8867 (111.836, -138.084) -> (111.831, -138.081)
  line L8868 (112.03, -138.191) -> (112.03, -138.191)
  line L8869 (114.578, -138.197) -> (114.578, -138.197)
  line L8870 (111.608, -138.003) -> (111.608, -138.003)
  line L8871 (112.216, -138.337) -> (112.212, -138.334)
  line L8872 (114.574, -138.193) -> (114.57, -138.191)
  line L8873 (113.24, -138.07) -> (113.091, -138.147)
  line L8874 (113.93, -137.964) -> (113.93, -137.964)
  line L8875 (114.148, -138.003) -> (113.93, -137.964)
  line L8876 (113.039, -138.175) -> (113.035, -138.178)
  line L8877 (114.366, -138.08) -> (114.158, -138.006)
  line L8878 (114.376, -138.084) -> (114.376, -138.084)
  line L8879 (111.613, -138.004) -> (111.608, -138.003)
  line L8880 (112.416, -138.577) -> (112.375, -138.513)
  line L8881 (112.501, -138.633) -> (112.437, -138.602)
  line L8882 (114.57, -138.191) -> (114.376, -138.084)
  line L8883 (114.158, -138.006) -> (114.153, -138.004)
  line L8884 (112.038, -138.197) -> (112.038, -138.197)
  line L8885 (113.699, -137.961) -> (113.693, -137.961)
  line L8886 (113.693, -137.961) -> (113.464, -137.996)
  line L8887 (112.694, -138.481) -> (112.626, -138.58)
  line L8888 (113.464, -137.996) -> (113.244, -138.068)
  line L8889 (113.699, -137.961) -> (113.699, -137.961)
  line L8890 (113.852, -137.963) -> (113.699, -137.961)
  line L8891 (114.376, -138.084) -> (114.371, -138.081)
  line L8892 (114.371, -138.081) -> (114.366, -138.08)
  line L8893 (114.781, -138.364) -> (114.756, -138.337)
  line L8894 (113.24, -138.07) -> (113.24, -138.07)
  line L8895 (113.93, -137.964) -> (113.925, -137.964)
  line L8896 (114.752, -138.334) -> (114.578, -138.197)
  line L8897 (111.618, -138.006) -> (111.613, -138.004)
  line L8898 (112.212, -138.334) -> (112.212, -138.334)
  line L8899 (114.57, -138.191) -> (114.57, -138.191)
  line L8900 (114.756, -138.337) -> (114.752, -138.334)
  line L8901 (113.244, -138.068) -> (113.24, -138.07)
  line L8902 (114.148, -138.003) -> (114.148, -138.003)
  line L8903 (114.158, -138.006) -> (114.158, -138.006)
  line L8904 (114.752, -138.334) -> (114.752, -138.334)
  line L8905 (114.366, -138.08) -> (114.366, -138.08)
  line L8906 (113.091, -138.147) -> (113.039, -138.175)
  line L8907 (114.578, -138.197) -> (114.574, -138.193)
  line L8908 (114.153, -138.004) -> (114.148, -138.003)
  line L8909 (114.892, -138.487) -> (114.781, -138.364)
  line L8910 (112.038, -138.197) -> (112.034, -138.193)
  line L8911 (116.099, -138.078) -> (115.888, -138.135)
  line L8912 (110.393, -138.254) -> (110.314, -138.314)
  line L8913 (111.159, -137.961) -> (111.153, -137.961)
  line L8914 (111.826, -138.08) -> (111.618, -138.006)
  line L8915 (112.372, -138.508) -> (112.352, -138.487)
  line L8916 (109.701, -138.364) -> (109.676, -138.337)
  line L8917 (109.832, -138.508) -> (109.812, -138.487)
  line L8918 (111.153, -137.961) -> (110.924, -137.996)
  line L8919 (113.035, -138.178) -> (113.035, -138.178)
  line L8920 (110.499, -138.175) -> (110.495, -138.178)
  line L8921 (109.672, -138.334) -> (109.672, -138.334)
  line L8922 (110.924, -137.996) -> (110.704, -138.068)
  line L8923 (111.836, -138.084) -> (111.836, -138.084)
  line L8924 (112.212, -138.334) -> (112.038, -138.197)
  line L8925 (110.154, -138.481) -> (110.086, -138.58)
  line L8926 (110.086, -138.58) -> (110.031, -138.625)
  line L8927 (111.385, -137.964) -> (111.312, -137.963)
  line L8928 (110.704, -138.068) -> (110.7, -138.07)
  line L8929 (110.495, -138.178) -> (110.495, -138.178)
  line L8930 (109.676, -138.337) -> (109.672, -138.334)
  line L8931 (110.551, -138.147) -> (110.499, -138.175)
  line L8932 (111.826, -138.08) -> (111.826, -138.08)
  line L8933 (109.498, -138.197) -> (109.498, -138.197)
  line L8934 (112.437, -138.602) -> (112.416, -138.577)
  line L8935 (110.314, -138.314) -> (110.154, -138.481)
  line L8936 (109.672, -138.334) -> (109.498, -138.197)
  line L8937 (110.7, -138.07) -> (110.551, -138.147)
  line L8938 (111.39, -137.964) -> (111.39, -137.964)
  line L8939 (112.03, -138.191) -> (111.836, -138.084)